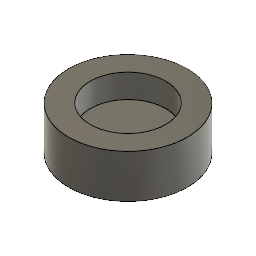
Cap thing (5) (Autodesk Fusion 360 design; units mm, degrees)
Autodesk Fusion 360 part; units mm, degrees
sketch "Sketch1" plane through (0, 0, 0) normal (0, 1, 0) x (1, 0, 0)
  circle A0 centre (0, 0) radius 1.9
  circle A1 centre (0, 0) radius 3
  dimension "d1" = 3.8
  dimension "d2" = 6
  measures "d1" diameter of A0
  measures "d2" diameter of A1
extrude "Extrude1" add sketch "Sketch1" along normal blind 3 contours A0 | A1
sketch "Sketch2" plane through (0, 3, 0) normal (0, 1, 0) x (-1, 0, 0)
  circle A0 centre (0, 0) radius 3
  circle A1 centre (0, 0) radius 1.9
  dimension "d5" = 3.8
  measures "d5" diameter of A1
extrude "Extrude2" cut sketch "Sketch2" against normal blind 2 contours A1
sketch "Sketch3" plane through (0, 1, 0) normal (0, 1, 0) x (-1, 0, 0)
  circle A0 centre (0, 0) radius 1.9
  circle A1 centre (0, 0) radius 2
  circle A2 centre (0, 0) radius 1.9
  dimension "d8" = 4
  measures "d8" diameter of A1
extrude "Extrude3" cut sketch "Sketch3" along normal blind 2.2
sketch "Sketch4" plane through (0, 1, 0) normal (0, 1, 0) x (-1, 0, 0)
  circle A0 centre (0, 0) radius 2
  circle A1 centre (0, 0) radius 2.1
  dimension "d11" = 4.2
  measures "d11" diameter of A1
extrude "Extrude4" cut sketch "Sketch4" along normal blind 2.8
sketch "Sketch5" plane through (0, 1, 0) normal (0, 1, 0) x (-1, 0, 0)
  circle A0 centre (0, 0) radius 2.1
  circle A1 centre (0, 0) radius 1.9
  dimension "d14" = 3.8
  measures "d14" diameter of A1
extrude "Extrude5" add sketch "Sketch5" along normal blind 2
sketch "Sketch6" plane through (0, 0, 0) normal (0, 0, 1) x (1, 0, 0)
  line L0 (-3.6792, 2.2002) -> (4.0444, 2.2002)
  line L1 (4.0444, 2.2002) -> (4.0444, 3.7157)
  line L2 (4.0444, 3.7157) -> (-3.2227, 3.7157)
  line L3 (-3.2227, 3.7157) -> (-3.2227, 2.2002)
extrude "Extrude6" cut sketch "Sketch6" along normal blind 4.5 and the other way blind 4.5
